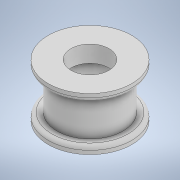
# Autodesk Inventor part: Roller
Saved by Autodesk Inventor 2022 (Build 260153000, 153)
## iProperties
Created: 2022-03-06
Part Number: Roller
Material: Genérico
Document SubType Name: Modeling
Designer: JK
Density: 1 g/cm^3
Appearance: Valor por defecto
Author: JK
Autodesk Inventor part; units mm, degrees
ref_plane "YZ Plane" through (0, 0, 0) normal (1, 0, 0) x (0, 1, 0)
ref_plane "XZ Plane" through (0, 0, 0) normal (0, 1, 0) x (-1, 0, 0)
ref_plane "XY Plane" through (0, 0, 0) normal (0, 0, 1) x (1, 0, 0)
sketch "Boceto1" plane through (0, 0, 0) normal (0, 1, 0) x (-1, 0, 0)
  circle A0 centre (0, 0) radius 8.125
  circle A1 centre (0, 0) radius 8.925
  dimension "d0" = 16.25
  dimension "d1" = 0.8
  constraints: 2 centre point, 2 coincident
  measures "d0" diameter of A0
  measures "d1" radial gap between concentric circles of A1 A0
extrude "Extrusión1" add sketch "Boceto1" along normal mid plane 10.3
sketch "Boceto2" plane through (0, 5.15, 0) normal (0, 1, 0) x (1, 0, 0)
  circle A0 centre (0, 0) radius 11.2887
  circle A1 centre (0, 0) radius 8.925 projected
  circle A2 centre (0, 0) radius 8.125 projected
  constraints: 1 centre point, 1 coincident
extrude "Extrusión2" add sketch "Boceto2" along normal blind 2 contours A0 | A1
fillet "Empalme1" radius 1 1 edges at (-11.2887, 5.15, 0)
mirror "Simetría1" about plane through (0, 0, 0) normal (0, 1, 0) of "Extrusión2", "Empalme1"
sketch "Boceto3" plane through (0, 7.15, 0) normal (0, 1, 0) x (1, 0, 0)
  circle A0 centre (0, 0) radius 8.125 projected
  circle A1 centre (0, 0) radius 5.125
  dimension "d7" = 10.25
  constraints: 1 centre point, 1 coincident
  measures "d7" diameter of A1
extrude "Extrusión3" add sketch "Boceto3" against normal blind 4.515
